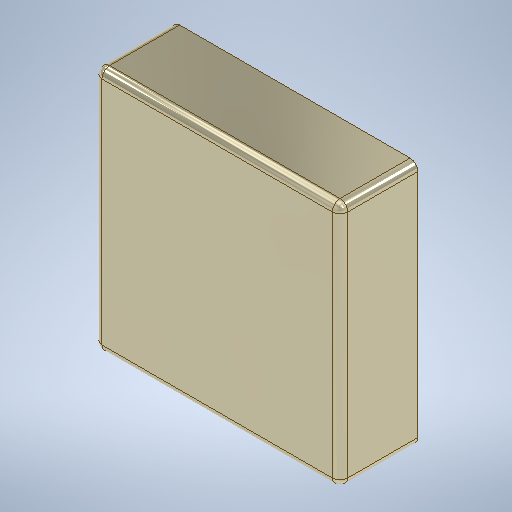
# Autodesk Inventor part: LimB_module
Saved by Autodesk Inventor 2025 (Build 290162000, 162)
## iProperties
Created: 2026-06-03
Part Number: LimB_module
Material: Brass
Document SubType Name: Modeling
Designer: rohan
Density: 8.49 g/cm^3
Appearance: Brass - Polished
Author: rohan
Autodesk Inventor part; units mm, degrees
ref_plane "YZ Plane" through (0, 0, 0) normal (1, 0, 0) x (0, 1, 0)
ref_plane "XZ Plane" through (0, 0, 0) normal (0, 1, 0) x (-1, 0, 0)
ref_plane "XY Plane" through (0, 0, 0) normal (0, 0, 1) x (1, 0, 0)
sketch "Sketch1" plane through (0, 0, 0) normal (0, 0, 1) x (1, 0, 0)
  line L0 (-10, -0.3003) -> (50, -0.3003)
  line L1 (50, -0.3003) -> (50, -60.3003)
  line L2 (50, -60.3003) -> (-10, -60.3003)
  line L3 (-10, -60.3003) -> (-10, -0.3003)
  line L4 (-11.6, 1.2997) -> (51.6, 1.2997)
  line L5 (51.6, 1.2997) -> (51.6, -61.9003)
  line L6 (51.6, -61.9003) -> (-11.6, -61.9003)
  line L7 (-11.6, -61.9003) -> (-11.6, 1.2997)
  point P0 (-10, -30.3003)
  point P1 (-11.6, -30.3003)
  dimension "d1" = 60
  dimension "d2" = 60
  dimension "d3" = 1.6
  dimension "d4" = 1.6
  dimension "d5" = 1.6
  dimension "d6" = 1.6
  constraints: 16 end point, 4 parallel, 2 horizontal, 2 midpoint, 2 perpendicular
  measures "d1" distance of L1.end L2.end
  measures "d2" distance of L0.end L1.end
  measures "d3" distance between parallel lines of L0 L4
  measures "d4" distance between parallel lines of L6 L2
  measures "d5" distance of point (-10, -30.3) point (-11.6, -30.3)
  measures "d6" distance between parallel lines of L5 L1
extrude "Extrusion1" add sketch "Sketch1" along normal blind 20 contours L0 L1 L2 L3 | L4 L5 L6 L7
sketch "Sketch2" plane through (0, 0, 0) normal (0, 0, -1) x (-1, 0, 0)
  line L0 (-50, -0.3003) -> (10, -0.3003)
  line L1 (10, -0.3003) -> (10, -60.3003)
  line L2 (10, -60.3003) -> (-50, -60.3003)
  line L3 (-50, -60.3003) -> (-50, -0.3003)
  line L4 (-51.6, 1.2997) -> (11.6, 1.2997) projected
  line L5 (11.6, -61.9003) -> (-51.6, -61.9003) projected
  line L6 (-51.6, -61.9003) -> (-51.6, 1.2997) projected
  line L7 (11.6, 1.2997) -> (11.6, -61.9003) projected
  point P0 (0, 0)
  dimension "d9" = 60
  dimension "d10" = 1.6
  dimension "d11" = 1.6
  dimension "d12" = 1.6
  dimension "d61" = 1.6
  constraints: 8 end point, 2 parallel, 1 horizontal, 1 perpendicular
  measures "d9" distance of L1.end L2.end
  measures "d10" distance between parallel lines of L0 L4
  measures "d11" distance between parallel lines of L5 L2
  measures "d12" distance between parallel lines of L6 L3
  measures "d61" distance between parallel lines of L7 L1
extrude "Extrusion2" cut sketch "Sketch2" against normal blind 18.4 contours L0 L1 L2 L3
sketch "Sketch3" plane through (-11.6, -61.9003, 0) normal (0, -1, 0) x (1, 0, 0)
  line L0 (57.6038, 13.4) -> (47.6038, 13.4)
  line L1 (47.6038, 13.4) -> (47.6038, 18.4)
  line L2 (47.6038, 18.4) -> (57.6038, 18.4)
  line L3 (57.6038, 18.4) -> (57.6038, 13.4)
  line L4 (0, 20) -> (63.2, 20) projected
  point P0 (11.6, 0)
  point P1 (52.6038, 18.4)
  dimension "d15" = 10
  dimension "d16" = 5
  dimension "d17" = 1.6
  constraints: 8 end point, 2 parallel, 1 horizontal, 1 midpoint, 1 perpendicular
  measures "d15" distance of L1.end L2.end
  measures "d16" distance of L0.end L1.end
  measures "d17" distance from line of L4 point (52.604, 18.4)
extrude "Extrusion3" cut sketch "Sketch3" against normal blind 18.4
fillet "Fillet1" radius 2 1 edges at (-11.6, -61.9003, 10)
fillet "Fillet2" radius 2 3 edges at (-11.6, 1.2997, 10) (51.6, 1.2997, 10) (51.6, -61.9003, 10)
fillet "Fillet3" radius 2 8 edges at (51.0142, -61.3145, 20) (51.6, -30.3003, 20) (51.0142, 0.7139, 20) (20, 1.2997, 20) (-11.0142, 0.7139, 20) (-11.6, -30.3003, 20) (-11.0142, -61.3145, 20) (20, -61.9003, 20)
sketch "Sketch4" plane through (-11.6, -59.9003, 0) normal (-1, 0, 0) x (0, 0, 1)
  line L0 (14.4, 37.5852) -> (18.4, 37.5852)
  line L1 (18.4, 37.5852) -> (18.4, 45.5852)
  line L2 (18.4, 45.5852) -> (14.4, 45.5852)
  line L3 (14.4, 45.5852) -> (14.4, 37.5852)
  line L4 (20, 0) -> (20, 59.2) projected
  point P0 (0, 59.9003)
  point P1 (18.4, 41.5852)
  dimension "d23" = 4
  dimension "d24" = 8
  dimension "d25" = 1.6
  constraints: 8 end point, 2 parallel, 1 horizontal, 1 midpoint, 1 perpendicular
  measures "d23" distance of L2.end L1.end
  measures "d24" distance of L1.end L0.end
  measures "d25" distance from line of L4 point (18.4, 41.585)
extrude "Extrusion4" cut sketch "Sketch4" against normal blind 18.4
sketch "Sketch5" plane through (0, 0, 18.4) normal (0, 0, -1) x (-1, 0, 0)
  point P0 (0, 0)
sketch "Sketch6" plane through (0, 0, 18.4) normal (0, 0, -1) x (-1, 0, 0)
  point P0 (0, 0)
fillet "Fillet4" radius 2 4 edges at (50, -0.3003, 9.2) (-10, -0.3003, 9.2) (-10, -60.3003, 9.2) (50, -60.3003, 9.2)
sketch "Sketch7" plane through (0, 0, 18.4) normal (0, 0, -1) x (-1, 0, 0)
  point P0 (0, 0)
sketch "Sketch8" plane through (0, 0, 18.4) normal (0, 0, -1) x (-1, 0, 0)
  circle A0 centre (-46.25, -4.0503) radius 2.6
  circle A1 centre (6.25, -56.5503) radius 2.6
  line L0 (-48, -0.3003) -> (8, -0.3003) projected
  line L1 (-50, -58.3003) -> (-50, -2.3003) projected
  line L2 (10, -2.3003) -> (10, -58.3003) projected
  line L3 (8, -60.3003) -> (-48, -60.3003) projected
  point P0 (0, 0)
  dimension "d30" = 5.2
  dimension "d31" = 5.2
  dimension "d32" = 3.75
  dimension "d33" = 3.75
  dimension "d34" = 3.75
  dimension "d35" = 3.75
  constraints: 2 centre point
  measures "d30" diameter of A0
  measures "d31" diameter of A1
  measures "d32" distance from line of A0.centre L0
  measures "d33" distance from line of L1 A0.centre
  measures "d34" distance from line of L2 A1.centre
  measures "d35" distance from line of L3 A1.centre
extrude "Extrusion5" add sketch "Sketch8" along normal up to surface (18.4 mm away)
sketch "Sketch9" plane through (46.25, -4.0503, 0) normal (0, 0, -1) x (-1, 0, 0)
  circle A0 centre (0, 0) radius 2.6 projected
  point P0 (46.25, 4.0503)
  constraints: 1 coincident
hole "Hole1" at (46.25, -4.0503, 0) direction (0, 0, 1) diameter 3.8 depth 6 tip angle 118
sketch "Sketch10" plane through (-6.25, -56.5503, 0) normal (0, 0, -1) x (-1, 0, 0)
  circle A0 centre (0, 0) radius 2.6 projected
  point P0 (-6.25, 56.5503)
  constraints: 1 coincident
hole "Hole2" at (-6.25, -56.5503, 0) direction (0, 0, 1) diameter 3.8 depth 6 tip angle 118
sketch "Sketch11" plane through (0, 0, 18.4) normal (0, 0, -1) x (-1, 0, 0)
  circle A0 centre (-9.4611, -3.3127) radius 1.25
  circle A1 centre (-9.4611, -18.5527) radius 1.25
  circle A2 centre (-31.0511, -3.3127) radius 1.25
  circle A3 centre (-31.0511, -18.5527) radius 1.25
  line L0 (-50, -58.3003) -> (-50, -2.3003) projected
  point P0 (0, 0)
  dimension "d54" = 2.5
  dimension "d55" = 2.5
  dimension "d56" = 2.5
  dimension "d57" = 2.5
  constraints: 4 centre point
  measures "d54" diameter of A0
  measures "d55" diameter of A1
  measures "d56" diameter of A2
  measures "d57" diameter of A3
extrude "Extrusion6" add sketch "Sketch11" along normal blind 8
body "Solid1"
